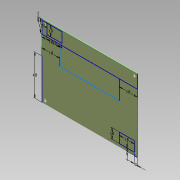
# Autodesk Inventor part: 基板
Saved by Autodesk Inventor 2017 (Build 210142000, 142)
## iProperties
Part Number: 基板
Material: 一般
Document SubType Name: Modeling
Designer: HISAAKI
Density: 1 g/cm^3
Appearance: 既定
Author: HISAAKI
Autodesk Inventor part; units mm, degrees
ref_plane "YZ Plane" through (0, 0, 0) normal (1, 0, 0) x (0, 1, 0)
ref_plane "XZ Plane" through (0, 0, 0) normal (0, 1, 0) x (-1, 0, 0)
ref_plane "XY Plane" through (0, 0, 0) normal (0, 0, 1) x (1, 0, 0)
sketch "スケッチ1" plane through (0, 0, 0) normal (0, 1, 0) x (-1, 0, 0)
  line L0 (0, 0) -> (95, 0)
  line L1 (95, 0) -> (95, -72)
  line L2 (95, -72) -> (0, -72)
  line L3 (0, -72) -> (0, 0)
  dimension "d0" = 95
  dimension "d1" = 72
  constraints: 8 end point, 2 parallel, 1 horizontal, 1 perpendicular
  measures "d0" distance of L1.end L2.end
  measures "d1" distance of L0.end L1.end
extrude "押し出し1" add sketch "スケッチ1" along normal blind 1
hole "穴1" at (-92, 1, -3) direction (0, -1, 0) diameter 3 end through all
hole "穴2" at (-92, 1, -69) direction (0, -1, 0) diameter 3 end through all
hole "穴3" at (-3, 1, -3) direction (0, -1, 0) diameter 3 end through all
hole "穴4" at (-3, 1, -69) direction (0, -1, 0) diameter 3 end through all
sketch "スケッチ2" plane through (0, 0, 0) normal (0, -1, 0) x (1, 0, 0)
  line L0 (-95, 0) -> (0, 0) projected
  line L1 (-95, 0) -> (-95, -1)
  line L2 (-95, -72) -> (-95, 0) projected
  line L3 (-95, -1) -> (-90, -1)
  line L4 (-90, -1) -> (-90, -11)
  line L5 (-90, -11) -> (-75, -11)
  line L6 (-75, -11) -> (-75, -1)
  line L7 (-75, -1) -> (-90, -1)
  line L8 (-95, 0) -> (-95, -13)
  line L9 (-95, -13) -> (-77, -13)
  line L10 (-95, -72) -> (-95, -32)
  line L11 (0, 0) -> (0, -13)
  line L12 (0, -13) -> (-18, -13)
  line L13 (-18, -13) -> (-77, -13)
  line L14 (-77, -13) -> (-77, -32)
  line L15 (-18, -13) -> (-18, -32)
  line L16 (-18, -32) -> (-77, -32)
  line L17 (0, 0) -> (0, -72) projected
  line L18 (0, -72) -> (-3, -72)
  line L19 (-3, -72) -> (-3, -69)
  line L20 (-3, -69) -> (-18, -69)
  line L21 (-18, -69) -> (-18, -59)
  line L22 (-18, -59) -> (-3, -59)
  circle A0 centre (-3, -69) radius 1.5 projected
  line L23 (-3, -59) -> (-3, -69)
  dimension "d40" = 1
  dimension "d41" = 5
  dimension "d42" = 10
  dimension "d43" = 15
  dimension "d44" = 13
  dimension "d45" = 18
  dimension "d46" = 40
  dimension "d47" = 18
  dimension "d48" = 18
  dimension "d49" = 3
  dimension "d50" = 3
  dimension "d51" = 15
  dimension "d52" = 10
  constraints: 42 end point, 8 perpendicular, 7 point on line, 2 collinear, 2 vertical, 1 horizontal, 1 parallel
  measures "d40" distance of L0.start L1.end
  measures "d41" distance of L1.end L3.end
  measures "d42" distance of L3.end L4.end
  measures "d43" distance of L4.end L5.end
  measures "d44" distance of L0.start L8.end
  measures "d45" distance of L8.end L9.end
  measures "d46" distance of L2.start L10.end
  measures "d47" distance of L10.end L14.end
  measures "d48" distance of L11.end L12.end
  measures "d49" distance of L17.end L18.end
  measures "d50" distance of L18.end L19.end
  measures "d51" distance of L19.end L20.end
  measures "d52" distance of L20.end L21.end
